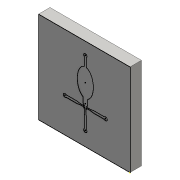
# Autodesk Inventor part: droplet-generator
Saved by Autodesk Inventor 2016 (Build 200138000, 138)
## iProperties
Created: 2018-10-05
Part Number: droplet-generator
Material: Genérico
Document SubType Name: Modeling
Designer: Joseahpacho
Density: 1 g/cm^3
Appearance: Valor por defecto
Author: Joseahpacho
Autodesk Inventor part; units mm, degrees
ref_plane "YZ Plane" through (0, 0, 0) normal (1, 0, 0) x (0, 1, 0)
ref_plane "XZ Plane" through (0, 0, 0) normal (0, 1, 0) x (-1, 0, 0)
ref_plane "XY Plane" through (0, 0, 0) normal (0, 0, 1) x (1, 0, 0)
sketch "Boceto1" plane through (0, 0, 0) normal (0, 1, 0) x (-1, 0, 0)
  arc A0 (19.363, 14.6519) -> (19.2523, 14.77) centre (19.0755, 14.4935) ccw
  arc A1 (19.9736, 14.77) -> (19.863, 14.6519) centre (20.1504, 14.4935) ccw
  ellipse E0 centre (19.613, 24.2247) end of major axis (19.613, 30.2556) minor radius 3.5091 (19.113, 30.1941) -> (18.6267, 18.4369) ccw
  arc A2 (18.6267, 16.2507) -> (19.2422, 15.3368) centre (19.613, 16.2507) ccw
  arc A3 (19.9837, 15.3368) -> (20.5992, 16.2507) centre (19.613, 16.2507) ccw
  line L0 (20.5992, 16.2507) -> (20.5992, 18.4369)
  line L1 (23.3999, 14.52) -> (21.7772, 14.77)
  line L2 (21.7772, 15.27) -> (23.3999, 15.52)
  line L3 (40, 0) -> (0, 0)
  line L4 (18.6267, 16.2507) -> (18.6267, 18.4369)
  ellipse E1 centre (19.613, 24.2247) end of major axis (19.613, 30.2556) minor radius 3.5091 (20.5992, 18.4369) -> (20.113, 30.1941) ccw
  line L5 (21.7772, 14.77) -> (19.9736, 14.77)
  line L6 (19.997, 15.27) -> (21.7772, 15.27)
  line L7 (19.997, 15.27) -> (19.9109, 15.27)
  line L8 (19.9109, 15.27) -> (19.9837, 15.3368)
  line L9 (19.2289, 15.27) -> (19.315, 15.27)
  line L10 (19.315, 15.27) -> (19.2422, 15.3368)
  arc A4 (27.9362, 14.52) -> (27.9362, 15.52) centre (28.4952, 15.02) ccw
  line L11 (23.3999, 15.52) -> (27.9362, 15.52)
  line L12 (23.3999, 14.52) -> (27.9362, 14.52)
  line L13 (15.8494, 15.52) -> (17.4722, 15.27)
  line L14 (17.4722, 14.77) -> (15.8494, 14.52)
  line L15 (17.4722, 15.27) -> (19.2757, 15.27)
  line L16 (19.2523, 14.77) -> (17.4722, 14.77)
  arc A5 (11.3132, 15.52) -> (11.3132, 14.52) centre (10.7541, 15.02) ccw
  line L17 (15.8494, 14.52) -> (11.3132, 14.52)
  line L18 (15.8494, 15.52) -> (11.3132, 15.52)
  line L19 (19.863, 12.8717) -> (20.113, 11.249)
  line L20 (19.113, 11.249) -> (19.363, 12.8717)
  line L21 (20.113, 11.249) -> (20.113, 6.7127)
  arc A6 (19.113, 6.7127) -> (20.113, 6.7127) centre (19.613, 6.1537) ccw
  line L22 (19.113, 11.249) -> (19.113, 6.7127)
  line L23 (19.363, 12.8717) -> (19.363, 14.6519)
  line L24 (19.863, 14.6519) -> (19.863, 12.8717)
  arc A7 (20.113, 33.9983) -> (19.113, 33.9983) centre (19.613, 34.5573) ccw
  line L25 (19.113, 30.1941) -> (19.113, 33.9983)
  line L26 (20.113, 30.1941) -> (20.113, 33.9983)
  line L27 (0, 0) -> (0, 40)
  line L28 (0, 40) -> (40, 40)
  line L29 (40, 40) -> (40, 0)
  constraints: 60 end point, 16 point on circle, 8 centre point, 2 horizontal, 2 perpendicular, 1 point on line, 1 vertical, 8 other
extrude "Extrusión1" add sketch "Boceto1" along normal blind 5 contours A0 L16 L14 L17 A5 L18 L13 L15 L9 L10 A2 L4 E0 L25 A7 L26 E1 L0 A3 L8 L7 L6 L2 L11 A4 L12 L1 L5 A1 L24 L19 L21 A6 L22 L20 L23 | L3 L27 L28 L29
extrude "Extrusión2" cut sketch "Boceto1" along normal blind 0.2 contours A0 L16 L14 L17 A5 L18 L13 L15 L9 L10 A2 L4 E0 L25 A7 L26 E1 L0 A3 L8 L7 L6 L2 L11 A4 L12 L1 L5 A1 L24 L19 L21 A6 L22 L20 L23
sketch "Boceto2" plane through (0, 0.2, 0) normal (0, -1, 0) x (1, 0, 0)
  arc A0 (-19.113, 33.9983) -> (-20.113, 33.9983) centre (-19.613, 34.5573) ccw projected
  arc A1 (-11.3132, 14.52) -> (-11.3132, 15.52) centre (-10.7541, 15.02) ccw projected
  arc A2 (-20.113, 6.7127) -> (-19.113, 6.7127) centre (-19.613, 6.1537) ccw projected
  arc A3 (-27.9362, 15.52) -> (-27.9362, 14.52) centre (-28.4952, 15.02) ccw projected
  circle A4 centre (-28.4952, 15.02) radius 0.35
  circle A5 centre (-19.613, 6.1537) radius 0.35
  circle A6 centre (-10.7541, 15.02) radius 0.35
  circle A7 centre (-19.613, 34.5573) radius 0.35
  point P0 (0, 0)
  dimension "d11" = 0.7
  dimension "d12" = 0.7
  dimension "d13" = 0.7
  dimension "d14" = 0.7
  constraints: 4 centre point, 4 coincident
  measures "d11" diameter of A4
  measures "d12" diameter of A5
  measures "d13" diameter of A6
  measures "d14" diameter of A7
extrude "Extrusión3" cut sketch "Boceto2" against normal through all
